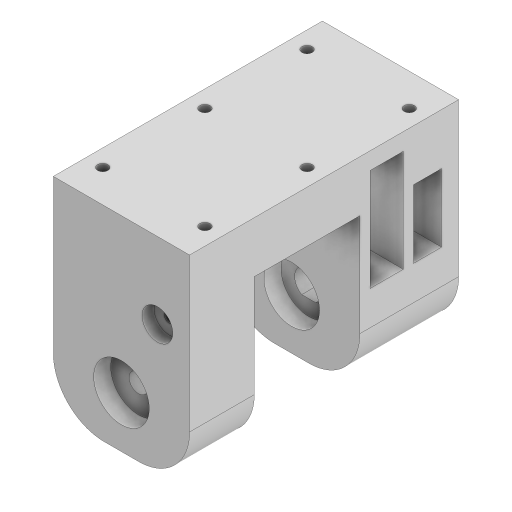
# Autodesk Inventor part: Gimbal_1
Saved by Autodesk Inventor 2023 (Build 270158000, 158)
## iProperties
Created: 2023-10-18
Part Number: Gimbal_1
Material: Generic
Document SubType Name: Modeling
Designer: MVeszpremi
Density: 1 g/cm^3
Appearance: Default
Author: MVeszpremi
Autodesk Inventor part; units mm, degrees
ref_plane "YZ Plane" through (0, 0, 0) normal (1, 0, 0) x (0, 1, 0)
ref_plane "XZ Plane" through (0, 0, 0) normal (0, 1, 0) x (-1, 0, 0)
ref_plane "XY Plane" through (0, 0, 0) normal (0, 0, 1) x (1, 0, 0)
sketch "Sketch1" plane through (0, 0, 0) normal (0, 1, 0) x (-1, 0, 0)
  line L0 (20, 34.5) -> (-20, 34.5)
  line L1 (-20, 34.5) -> (-20, 15.5)
  line L2 (-20, 15.5) -> (20, 15.5)
  line L3 (20, 15.5) -> (20, 34.5)
  line L4 (20, -15.5) -> (-20, -15.5)
  line L5 (-20, -15.5) -> (-20, -44.5)
  line L6 (-20, -44.5) -> (20, -44.5)
  line L7 (20, -44.5) -> (20, -15.5)
  point P0 (0, 0)
  dimension "d0" = 31
  dimension "d1" = 19
  dimension "d2" = 40
  dimension "d3" = 20
  dimension "d4" = 29
  dimension "d50" = 15.5
  constraints: 16 end point, 4 parallel, 2 horizontal, 2 perpendicular, 2 point on line
  measures "d0" distance between parallel lines of L4 L2
  measures "d1" distance of L2.end L0.start
  measures "d2" distance of L0.start L0.end
  measures "d3" distance from line of L3 point (0, 0)
  measures "d4" distance of L6.end L4.start
  measures "d50" distance from line of L2 point (0, 0)
sketch "Sketch1 outline for Extrusion1" plane through (0, 0, 0) normal (0, 1, 0) x (-1, 0, 0)
  line L0 (20, -15.5) -> (-20, -15.5)
  line L1 (20, -44.5) -> (20, -15.5)
  line L2 (-20, -44.5) -> (20, -44.5)
  line L3 (-20, -15.5) -> (-20, -44.5)
  line L4 (20, 34.5) -> (-20, 34.5)
  line L5 (20, 15.5) -> (20, 34.5)
  line L6 (-20, 15.5) -> (20, 15.5)
  line L7 (-20, 34.5) -> (-20, 15.5)
extrude "Extrusion1" add sketch "Sketch1 outline for Extrusion1" along normal blind 45
sketch "Sketch2" plane through (20, 0, -44.5) normal (0, 0, -1) x (-1, 0, 0)
  circle A0 centre (20, 15) radius 8.125
  line L0 (0, 0) -> (40, 0) projected
  circle A1 centre (20, 15) radius 2.75
  point P0 (20, 0)
  point P1 (20, 0)
  dimension "d7" = 16.25
  dimension "d8" = 15
  dimension "d9" = 5.5
  constraints: 2 centre point, 1 coincident, 1 midpoint
  measures "d7" diameter of A0
  measures "d8" distance of point (20, 0) A0.centre
  measures "d9" diameter of A1
sketch "Sketch2 outline for Extrusion2" plane through (20, 0, -44.5) normal (0, 0, -1) x (-1, 0, 0)
  circle A0 centre (20, 15) radius 2.75
extrude "Extrusion2" cut sketch "Sketch2 outline for Extrusion2" against normal blind 274.75
sketch "Sketch3" plane through (0, 45, 0) normal (0, 1, 0) x (1, 0, 0)
  line L0 (20, -34.5) -> (20, -15.5) projected
  line L1 (-20, 44.5) -> (-20, 15.5) projected
  line L2 (20, -34.5) -> (-20, -34.5)
  line L3 (-20, -34.5) -> (-20, 44.5)
  line L4 (-20, 44.5) -> (20, 44.5)
  line L5 (20, 44.5) -> (20, -34.5)
  point P0 (0, 0)
  constraints: 8 end point, 2 parallel, 1 horizontal, 1 perpendicular
sketch "Sketch3 outline for Extrusion3" plane through (0, 45, 0) normal (0, 1, 0) x (1, 0, 0)
  line L0 (-20, -34.5) -> (20, -34.5)
  line L1 (-20, 15.5) -> (-20, -34.5)
  line L2 (-20, 44.5) -> (-20, 15.5)
  line L3 (20, 44.5) -> (-20, 44.5)
  line L4 (20, -15.5) -> (20, 44.5)
  line L5 (20, -34.5) -> (20, -15.5)
extrude "Extrusion3" add sketch "Sketch3 outline for Extrusion3" along normal blind 15
sketch "Sketch4" plane through (-20, 0, -44.5) normal (-1, 0, 0) x (0, 0, 1)
  line L0 (5, 55) -> (26, 55)
  line L1 (26, 55) -> (26, 25)
  line L2 (26, 25) -> (5, 25)
  line L3 (5, 25) -> (5, 55)
  line L4 (0, 0) -> (0, 60) projected
  line L5 (29, 0) -> (29, 45) projected
  line L6 (0, 60) -> (79, 60) projected
  line L7 (0, 0) -> (29, 0) projected
  line L8 (13.25, 55) -> (16.25, 55)
  line L9 (16.25, 55) -> (16.25, 25)
  line L10 (16.25, 25) -> (13.25, 25)
  line L11 (13.25, 25) -> (13.25, 55)
  line L12 (5, 55) -> (13.25, 55)
  line L13 (13.25, 45) -> (5, 45)
  point P0 (44.5, 0)
  dimension "d14" = 5
  dimension "d15" = 3
  dimension "d16" = 5
  dimension "d18" = 3
  dimension "d19" = 9.75
  dimension "d45" = 25
  constraints: 20 end point, 6 point on line, 4 parallel, 4 perpendicular, 2 horizontal
  measures "d14" distance between parallel lines of L4 L3
  measures "d15" distance between parallel lines of L5 L1
  measures "d16" distance between parallel lines of L6 L0
  measures "d18" distance between parallel lines of L9 L11
  measures "d19" distance between parallel lines of L1 L9
  measures "d45" distance between parallel lines of L7 L2
sketch "Sketch4 outline for Extrusion4" plane through (-20, 0, -44.5) normal (-1, 0, 0) x (0, 0, 1)
  line L0 (26, 25) -> (26, 55)
  line L1 (16.25, 25) -> (26, 25)
  line L2 (16.25, 55) -> (16.25, 25)
  line L3 (26, 55) -> (16.25, 55)
  line L4 (13.25, 45) -> (5, 45)
  line L5 (13.25, 25) -> (13.25, 45)
  line L6 (5, 25) -> (13.25, 25)
  line L7 (5, 45) -> (5, 25)
extrude "Extrusion4" cut sketch "Sketch4 outline for Extrusion4" against normal blind 100
sketch "Sketch5" plane through (20, 0, -44.5) normal (0, 0, -1) x (-1, 0, 0)
  circle A0 centre (20, 15) radius 2.75
  circle A1 centre (20, 15) radius 4.15
  line L0 (17.935418, 11.4) -> (22.064582, 11.4)
  point P0 (20, 0)
  dimension "d22" = 8.3
  dimension "d24" = 3.6
  constraints: 2 end point, 2 point on circle, 1 centre point, 1 coincident, 1 horizontal
  measures "d22" diameter of A1
  measures "d24" distance from line of L0 A1.centre
sketch "Sketch5 outline for Extrusion5" plane through (20, 0, -44.5) normal (0, 0, -1) x (-1, 0, 0)
  line L0 (17.935418, 11.4) -> (22.064582, 11.4)
  arc A0 (22.064582, 11.4) -> (17.935418, 11.4) centre (20, 15) ccw
  circle A1 centre (20, 15) radius 2.75
extrude "Extrusion5" cut sketch "Sketch5 outline for Extrusion5" against normal blind 25
sketch "Sketch6" plane through (20, 0, -44.5) normal (0, 0, -1) x (-1, 0, 0)
  line L0 (16.375, 9.5) -> (23.625, 9.5)
  line L1 (23.625, 9.5) -> (23.625, 6)
  line L2 (23.625, 6) -> (16.375, 6)
  line L3 (16.375, 6) -> (16.375, 9.5)
  line L4 (0, 0) -> (40, 0) projected
  circle A0 centre (20, 15) radius 2.75 projected
  point P0 (20, 0)
  point P1 (20, 0)
  dimension "d27" = 3.5
  dimension "d28" = 7.25
  dimension "d29" = 3.625
  dimension "d30" = 5.5
  constraints: 8 end point, 2 parallel, 1 horizontal, 1 midpoint, 1 perpendicular
  measures "d27" distance between parallel lines of L2 L0
  measures "d28" distance of L0.start L0.end
  measures "d29" horizontal distance of point (20, 0) L2.end
  measures "d30" distance from line of A0.centre L0
sketch "Sketch6 outline for Extrusion6" plane through (20, 0, -44.5) normal (0, 0, -1) x (-1, 0, 0)
  line L0 (16.375, 9.5) -> (16.375, 6)
  line L1 (23.625, 9.5) -> (16.375, 9.5)
  line L2 (23.625, 6) -> (23.625, 9.5)
  line L3 (16.375, 6) -> (23.625, 6)
extrude "Extrusion6" cut sketch "Sketch6 outline for Extrusion6" against normal blind 23
sketch "Sketch7" plane through (0, 0, 0) normal (0, -1, 0) x (1, 0, 0)
  circle A0 centre (0, -37.5) radius 2
  point P0 (0, 0)
  dimension "d33" = 4
  dimension "d34" = 37.5
  constraints: 1 centre point
  measures "d33" diameter of A0
  measures "d34" distance of point (0, 0) A0.centre
sketch "Sketch7 outline for Extrusion7" plane through (0, 0, 0) normal (0, -1, 0) x (1, 0, 0)
  circle A0 centre (0, -37.5) radius 2
extrude "Extrusion7" cut sketch "Sketch7 outline for Extrusion7" against normal blind 15.5
sketch "Sketch8" plane through (-20, 0, -15.5) normal (0, 0, 1) x (1, 0, 0)
  circle A0 centre (20, 15) radius 2.75 projected
  circle A1 centre (20, 15) radius 8.15
  point P0 (20, 0)
  dimension "d37" = 16.3
  constraints: 1 centre point, 1 coincident
  measures "d37" diameter of A1
sketch "Sketch8 outline for Extrusion8" plane through (-20, 0, -15.5) normal (0, 0, 1) x (1, 0, 0)
  circle A0 centre (20, 15) radius 8.15
  circle A1 centre (20, 15) radius 2.75
extrude "Extrusion8" cut sketch "Sketch8 outline for Extrusion8" against normal blind 5
sketch "Sketch9" plane through (-20, 0, 34.5) normal (0, 0, 1) x (1, 0, 0)
  circle A0 centre (20, 15) radius 2.75 projected
  circle A1 centre (20, 15) radius 8.15
  point P0 (20, 0)
  constraints: 1 centre point, 1 coincident
sketch "Sketch9 outline for Extrusion9" plane through (-20, 0, 34.5) normal (0, 0, 1) x (1, 0, 0)
  circle A0 centre (20, 15) radius 8.15
  circle A1 centre (20, 15) radius 2.75
extrude "Extrusion9" cut sketch "Sketch9 outline for Extrusion9" against normal blind 5
sketch "Sketch10" plane through (20, 0, 15.5) normal (0, 0, -1) x (-1, 0, 0)
  circle A0 centre (20, 15) radius 2.75 projected
  circle A1 centre (20, 15) radius 8.15
  point P0 (20, 0)
  constraints: 1 centre point, 1 coincident
sketch "Sketch10 outline for Extrusion10" plane through (20, 0, 15.5) normal (0, 0, -1) x (-1, 0, 0)
  circle A0 centre (20, 15) radius 8.15
  circle A1 centre (20, 15) radius 2.75
extrude "Extrusion10" cut sketch "Sketch10 outline for Extrusion10" against normal blind 5
fillet "Fillet1" radius 15 4 edges at (-20, 0, -30) (-20, 0, 25) (20, 0, 25) (20, 0, -30)
sketch "Sketch11" plane through (0, 60, 0) normal (0, 1, 0) x (1, 0, 0)
  line L0 (-15, -25) -> (15, -25)
  line L1 (15, -25) -> (15, 35)
  line L2 (15, 35) -> (-15, 35)
  line L3 (-15, 35) -> (-15, -25)
  circle A0 centre (-15, -25) radius 1.5
  circle A1 centre (-15, 35) radius 1.5
  circle A2 centre (15, 35) radius 1.5
  circle A3 centre (15, -25) radius 1.5
  circle A4 centre (-15, 5) radius 1.5
  circle A5 centre (15, 5) radius 1.5
  point P0 (0, 0)
  dimension "d46" = 60
  dimension "d47" = 30
  dimension "d48" = 15
  dimension "d49" = 25
  dimension "d51" = 3
  dimension "d52" = 3
  dimension "d53" = 3
  dimension "d54" = 3
  dimension "d55" = 3
  dimension "d56" = 3
  constraints: 8 end point, 6 centre point, 4 coincident, 2 midpoint, 2 parallel, 1 horizontal, 1 perpendicular
  measures "d46" distance of L2.end L0.start
  measures "d47" distance of L0.start L0.end
  measures "d48" distance from line of L3 point (0, 0)
  measures "d49" distance from line of L0 point (0, 0)
  measures "d51" diameter of A0
  measures "d52" diameter of A1
  measures "d53" diameter of A2
  measures "d54" diameter of A3
  measures "d55" diameter of A4
  measures "d56" diameter of A5
sketch "Sketch11 outline for Extrusion11" plane through (0, 60, 0) normal (0, 1, 0) x (1, 0, 0)
  circle A0 centre (-15, 35) radius 1.5
  circle A1 centre (15, -25) radius 1.5
  circle A2 centre (15, 5) radius 1.5
  circle A3 centre (-15, -25) radius 1.5
  circle A4 centre (15, 35) radius 1.5
  circle A5 centre (-15, 5) radius 1.5
extrude "Extrusion11" cut sketch "Sketch11 outline for Extrusion11" against normal blind 15
sketch "Sketch12" plane through (20, 60, -44.5) normal (0, 0, -1) x (-1, 0, 0)
  arc A0 (22.064582, -48.6) -> (17.935418, -48.6) centre (20, -45) ccw
  circle A1 centre (20, -45) radius 4.15
  point P0 (20, -60)
  point P1 (17.935418, -48.6)
  constraints: 1 centre point, 1 coincident
sketch "Sketch12 outline for Extrusion12" plane through (20, 60, -44.5) normal (0, 0, -1) x (-1, 0, 0)
  arc A0 (17.935418, -48.6) -> (22.064582, -48.6) centre (20, -45) ccw
  arc A1 (22.064582, -48.6) -> (17.935418, -48.6) centre (20, -45) ccw
extrude "Extrusion12" cut sketch "Sketch12 outline for Extrusion12" against normal blind 2
sketch "Sketch13" plane through (20, 60, -44.5) normal (0, 0, -1) x (-1, 0, 0)
  arc A0 (22.064582, -48.6) -> (17.935418, -48.6) centre (20, -45) ccw
  circle A1 centre (20, -45) radius 10
  line L0 (20, -35) -> (40, -35)
  line L1 (40, -35) -> (0, -35)
  line L2 (0, -45) -> (0, 0)
  circle A2 centre (20, -45) radius 4.15
  arc A3 (0, -45) -> (15, -60) centre (15, -45) ccw
  line L3 (15, -60) -> (25, -60)
  arc A4 (25, -60) -> (40, -45) centre (25, -45) ccw
  line L4 (40, -45) -> (40, 0)
  line L5 (0, 0) -> (40, 0)
  line L6 (0, -45) -> (0, 0)
  line L7 (23.625, -50.5) -> (23.625, -54)
  line L8 (23.625, -54) -> (16.375, -54)
  line L9 (16.375, -54) -> (16.375, -50.5)
  line L10 (16.375, -50.5) -> (23.625, -50.5)
  circle A5 centre (20, -45) radius 18
  point P0 (20, -60)
  point P1 (40, -35)
  point P2 (17.935418, -48.6)
  point P3 (7.6, -58.047605)
  point P4 (34.96663, -35)
  point P5 (32.4, -58.047605)
  dimension "d61" = 20
  dimension "d64" = 36
  constraints: 4 end point, 2 coincident, 2 point on line, 1 centre point, 1 horizontal, 3 other
  measures "d64" diameter of A5
sketch "Sketch13 outline for Extrusion13" plane through (20, 60, -44.5) normal (0, 0, -1) x (-1, 0, 0)
  circle A0 centre (20, -45) radius 4.15
  line L0 (23.625, -50.5) -> (16.375, -50.5)
  line L1 (23.625, -54) -> (23.625, -50.5)
  line L2 (16.375, -54) -> (23.625, -54)
  line L3 (16.375, -50.5) -> (16.375, -54)
  arc A1 (32.4, -58.047605) -> (7.6, -58.047605) centre (20, -45) ccw
  arc A2 (25, -60) -> (32.4, -58.047605) centre (25, -45) ccw
  arc A3 (7.6, -58.047605) -> (15, -60) centre (15, -45) ccw
  line L4 (15, -60) -> (25, -60)
  circle A4 centre (20, -45) radius 10
extrude "Extrusion13" cut sketch "Sketch13 outline for Extrusion13" against normal blind 1.5
sketch "Sketch14" plane through (-20, 60, 34.5) normal (0, 0, 1) x (1, 0, 0)
  circle A0 centre (30.565457, -22.342305) radius 4.5
  circle A1 centre (20, -45) radius 2.75
  circle A2 centre (30.565457, -22.342305) radius 1.5
  line L0 (20, -45) -> (20, 2.624244)
  line L1 (20, 2.624244) -> (20, -45)
  line L2 (30.565457, -22.342305) -> (20, -45)
  point P0 (20, -60)
  dimension "d65" = 25
  dimension "d66" = 9
  dimension "d67" = 3
  dimension "d72" = 25
  constraints: 6 end point, 2 centre point, 1 coincident, 1 collinear, 1 vertical
  measures "d65" distance of A0.centre L0.start
  measures "d66" diameter of A0
  measures "d67" diameter of A2
  measures "d72" angle of L2 L0
sketch "Sketch14 outline for Extrusion14" plane through (-20, 60, 34.5) normal (0, 0, 1) x (1, 0, 0)
  circle A0 centre (30.565457, -22.342305) radius 1.5
extrude "Extrusion14" cut sketch "Sketch14 outline for Extrusion14" against normal blind 10
sketch "Sketch14 outline for Extrusion15" plane through (-20, 60, 34.5) normal (0, 0, 1) x (1, 0, 0)
  circle A0 centre (30.565457, -22.342305) radius 4.5
  circle A1 centre (30.565457, -22.342305) radius 1.5
extrude "Extrusion15" cut sketch "Sketch14 outline for Extrusion15" against normal blind 3.5
body "Solid1"
